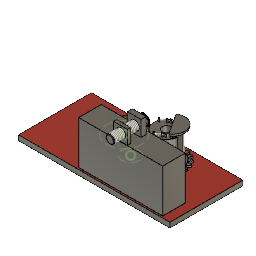
cambio de broca v1 (Autodesk Fusion 360 design; units mm, degrees)
description: Spur Gear; Module: 1.0; Num Teeth: 20; Pressure Angle: 25.0; Backlash: 0.00 mm
description: Spur Gear; Module: 1.0; Num Teeth: 10; Pressure Angle: 25.0; Backlash: 0.00 mm
Autodesk Fusion 360 part; units mm, degrees
(part 1 of 4)
sketch "Boceto1" plane through (0, 0, 0) normal (0, 0, 1) x (1, 0, 0) in component "Spur Gear (20 teeth)"
  circle A0 centre (0, 0) radius 8.7492
  circle A1 centre (0, 0) radius 2.5
extrude "Extruir1" add sketch "Boceto1" along normal blind 1 contours A0 picked at (6.63356, -0.434667) makes body 1 in component "Spur Gear (20 teeth)"
sketch "Boceto2" plane through (0, 0, 0) normal (0, 0, 1) x (1, 0, 0) in component "Spur Gear (20 teeth)"
  spline S0 degree 5 poles (9.009769, -0.981552) (9.015434, -0.98215) (9.026773, -0.983183) (9.043806, -0.984243) (9.066562, -0.984722) (9.095076, -0.984038) (9.123646, -0.982417) (9.152257, -0.980201) (9.1809, -0.977648) (9.209567, -0.974857) (9.238252, -0.971824) (9.266955, -0.968481) (9.295673, -0.964741) (9.324406, -0.960542) (9.353151, -0.955881) (9.381905, -0.950792) (9.410667, -0.945328) (9.439434, -0.939546) (9.468204, -0.933488) (9.496975, -0.927167) (9.525745, -0.920582) (9.554514, -0.913723) (9.583281, -0.906574) (9.612044, -0.899129) (9.640803, -0.891392) (9.669556, -0.883371) (9.698301, -0.875079) (9.727038, -0.86653) (9.755765, -0.857732) (9.784482, -0.848691) (9.813187, -0.839407) (9.84188, -0.829881) (9.870559, -0.820113) (9.899223, -0.810103) (9.927872, -0.799853) (9.956505, -0.789368) (9.985121, -0.778652) (10.013718, -0.767708) (10.042297, -0.756541) (10.070855, -0.745151) (10.099393, -0.733542) (10.127909, -0.721715) (10.156403, -0.709671) (10.184874, -0.697411) (10.213321, -0.684937) (10.241743, -0.672252) (10.270139, -0.659357) (10.298509, -0.646255) (10.326852, -0.632947) (10.355167, -0.619434) (10.383453, -0.605718) (10.41171, -0.591801) (10.439937, -0.577684) (10.468133, -0.563368) (10.496297, -0.548854) (10.524429, -0.534145) (10.552528, -0.51924) (10.580593, -0.504142) (10.608623, -0.488851) (10.636619, -0.47337) (10.664578, -0.457698) (10.692501, -0.441837) (10.720388, -0.425788) (10.748236, -0.409552) (10.776046, -0.393131) (10.803816, -0.376525) (10.831546, -0.359736) (10.859235, -0.342764) (10.886882, -0.325611) (10.914488, -0.308276) (10.942051, -0.290762) (10.964068, -0.276607) (10.980562, -0.26591) (10.991549, -0.258743) (10.99704, -0.25515) knots 0 0 0 0 0 0 0.01428571 0.02857143 0.04285714 0.05714286 0.07142857 0.08571429 0.1 0.11428571 0.12857143 0.14285714 0.15714286 0.17142857 0.18571429 0.2 0.21428571 0.22857143 0.24285714 0.25714286 0.27142857 0.28571429 0.3 0.31428571 0.32857143 0.34285714 0.35714286 0.37142857 0.38571429 0.4 0.41428571 0.42857143 0.44285714 0.45714286 0.47142857 0.48571429 0.5 0.51428571 0.52857143 0.54285714 0.55714286 0.57142857 0.58571429 0.6 0.61428571 0.62857143 0.64285714 0.65714286 0.67142857 0.68571429 0.7 0.71428571 0.72857143 0.74285714 0.75714286 0.77142857 0.78571429 0.8 0.81428571 0.82857143 0.84285714 0.85714286 0.87142857 0.88571429 0.9 0.91428571 0.92857143 0.94285714 0.95714286 0.97142857 0.98571429 1 1 1 1 1 1
  spline S1 degree 5 poles (9.009769, 0.981552) (9.015434, 0.98215) (9.026773, 0.983183) (9.043806, 0.984243) (9.066562, 0.984722) (9.095076, 0.984038) (9.123646, 0.982417) (9.152257, 0.980201) (9.1809, 0.977648) (9.209567, 0.974857) (9.238252, 0.971824) (9.266955, 0.968481) (9.295673, 0.964741) (9.324406, 0.960542) (9.353151, 0.955881) (9.381905, 0.950792) (9.410667, 0.945328) (9.439434, 0.939546) (9.468204, 0.933488) (9.496975, 0.927167) (9.525745, 0.920582) (9.554514, 0.913723) (9.583281, 0.906574) (9.612044, 0.899129) (9.640803, 0.891392) (9.669556, 0.883371) (9.698301, 0.875079) (9.727038, 0.86653) (9.755765, 0.857732) (9.784482, 0.848691) (9.813187, 0.839407) (9.84188, 0.829881) (9.870559, 0.820113) (9.899223, 0.810103) (9.927872, 0.799853) (9.956505, 0.789368) (9.985121, 0.778652) (10.013718, 0.767708) (10.042297, 0.756541) (10.070855, 0.745151) (10.099393, 0.733542) (10.127909, 0.721715) (10.156403, 0.709671) (10.184874, 0.697411) (10.213321, 0.684937) (10.241743, 0.672252) (10.270139, 0.659357) (10.298509, 0.646255) (10.326852, 0.632947) (10.355167, 0.619434) (10.383453, 0.605718) (10.41171, 0.591801) (10.439937, 0.577684) (10.468133, 0.563368) (10.496297, 0.548854) (10.524429, 0.534145) (10.552528, 0.51924) (10.580593, 0.504142) (10.608623, 0.488851) (10.636619, 0.47337) (10.664578, 0.457698) (10.692501, 0.441837) (10.720388, 0.425788) (10.748236, 0.409552) (10.776046, 0.393131) (10.803816, 0.376525) (10.831546, 0.359736) (10.859235, 0.342764) (10.886882, 0.325611) (10.914488, 0.308276) (10.942051, 0.290762) (10.964068, 0.276607) (10.980562, 0.26591) (10.991549, 0.258743) (10.99704, 0.25515) knots 0 0 0 0 0 0 0.01428571 0.02857143 0.04285714 0.05714286 0.07142857 0.08571429 0.1 0.11428571 0.12857143 0.14285714 0.15714286 0.17142857 0.18571429 0.2 0.21428571 0.22857143 0.24285714 0.25714286 0.27142857 0.28571429 0.3 0.31428571 0.32857143 0.34285714 0.35714286 0.37142857 0.38571429 0.4 0.41428571 0.42857143 0.44285714 0.45714286 0.47142857 0.48571429 0.5 0.51428571 0.52857143 0.54285714 0.55714286 0.57142857 0.58571429 0.6 0.61428571 0.62857143 0.64285714 0.65714286 0.67142857 0.68571429 0.7 0.71428571 0.72857143 0.74285714 0.75714286 0.77142857 0.78571429 0.8 0.81428571 0.82857143 0.84285714 0.85714286 0.87142857 0.88571429 0.9 0.91428571 0.92857143 0.94285714 0.95714286 0.97142857 0.98571429 1 1 1 1 1 1
  arc A0 (10.99704, -0.25515) -> (10.99704, 0.25515) centre (0, 0) ccw
  line L0 (8.687796, -0.947559) -> (9.009769, -0.981552)
  line L1 (8.687796, 0.947559) -> (9.009769, 0.981552)
  line L2 (8.687796, -0.947559) -> (8.687796, 0.947559)
  point P0 (9.149052, -0.980379)
  point P1 (9.289749, -0.965437)
  point P2 (9.431291, -0.941141)
  point P3 (9.573428, -0.908982)
  point P4 (9.715981, -0.869786)
  point P5 (9.858805, -0.824084)
  point P6 (10.00177, -0.772251)
  point P7 (10.144756, -0.714565)
  point P8 (10.28765, -0.651241)
  point P9 (10.430344, -0.582452)
  point P10 (10.572732, -0.508339)
  point P11 (10.714711, -0.42902)
  point P12 (10.856181, -0.344594)
  point P13 (9.149052, 0.980379)
  point P14 (9.289749, 0.965437)
  point P15 (9.431291, 0.941141)
  point P16 (9.573428, 0.908982)
  point P17 (9.715981, 0.869786)
  point P18 (9.858805, 0.824084)
  point P19 (10.00177, 0.772251)
  point P20 (10.144756, 0.714565)
  point P21 (10.28765, 0.651241)
  point P22 (10.430344, 0.582452)
  point P23 (10.572732, 0.508339)
  point P24 (10.714711, 0.42902)
  point P25 (10.856181, 0.344594)
extrude "Extruir2" add sketch "Boceto2" along normal blind 1 contours S0 S1 A0 L0 L1 L2 picked at (9.651017, 0.26303) bodies 1 in component "Spur Gear (20 teeth)"
pattern_circular "Patrón C1" count 20 over 360 about axis through (0, 0, 0) along (0, 0, 1) of "Extruir2" in component "Spur Gear (20 teeth)"
sketch "Boceto3" plane through (0, 0, 0) normal (0, 0, 1) x (1, 0, 0) in component "Spur Gear (20 teeth)"
  circle A0 centre (0, 0) radius 10 construction
sketch "Boceto1 (2)" plane through (0, 0, 0) normal (0, 0, 1) x (1, 0, 0) in component "Spur Gear (20 teeth) (1)"
  circle A0 centre (0, 0) radius 8.652617
  circle A1 centre (0, 0) radius 2.130605
extrude "Extruir1'" add sketch "Boceto1 (2)" along normal blind 1 separate body contours A0 picked at (6.446398, -0.429869) makes body 2 in component "Spur Gear (20 teeth) (1)"
sketch "Boceto2 (2)" plane through (0, 0, 0) normal (0, 0, 1) x (1, 0, 0) in component "Spur Gear (20 teeth) (1)"
  spline S0 degree 5 poles (9.009769, -0.981552) (9.015434, -0.98215) (9.026773, -0.983183) (9.043806, -0.984243) (9.066562, -0.984722) (9.095076, -0.984038) (9.123646, -0.982417) (9.152257, -0.980201) (9.1809, -0.977648) (9.209567, -0.974857) (9.238252, -0.971824) (9.266955, -0.968481) (9.295673, -0.964741) (9.324406, -0.960542) (9.353151, -0.955881) (9.381905, -0.950792) (9.410667, -0.945328) (9.439434, -0.939546) (9.468204, -0.933488) (9.496975, -0.927167) (9.525745, -0.920582) (9.554514, -0.913723) (9.583281, -0.906574) (9.612044, -0.899129) (9.640803, -0.891392) (9.669556, -0.883371) (9.698301, -0.875079) (9.727038, -0.86653) (9.755765, -0.857732) (9.784482, -0.848691) (9.813187, -0.839407) (9.84188, -0.829881) (9.870559, -0.820113) (9.899223, -0.810103) (9.927872, -0.799853) (9.956505, -0.789368) (9.985121, -0.778652) (10.013718, -0.767708) (10.042297, -0.756541) (10.070855, -0.745151) (10.099393, -0.733542) (10.127909, -0.721715) (10.156403, -0.709671) (10.184874, -0.697411) (10.213321, -0.684937) (10.241743, -0.672252) (10.270139, -0.659357) (10.298509, -0.646255) (10.326852, -0.632947) (10.355167, -0.619434) (10.383453, -0.605718) (10.41171, -0.591801) (10.439937, -0.577684) (10.468133, -0.563368) (10.496297, -0.548854) (10.524429, -0.534145) (10.552528, -0.51924) (10.580593, -0.504142) (10.608623, -0.488851) (10.636619, -0.47337) (10.664578, -0.457698) (10.692501, -0.441837) (10.720388, -0.425788) (10.748236, -0.409552) (10.776046, -0.393131) (10.803816, -0.376525) (10.831546, -0.359736) (10.859235, -0.342764) (10.886882, -0.325611) (10.914488, -0.308276) (10.942051, -0.290762) (10.964068, -0.276607) (10.980562, -0.26591) (10.991549, -0.258743) (10.99704, -0.25515) knots 0 0 0 0 0 0 0.01428571 0.02857143 0.04285714 0.05714286 0.07142857 0.08571429 0.1 0.11428571 0.12857143 0.14285714 0.15714286 0.17142857 0.18571429 0.2 0.21428571 0.22857143 0.24285714 0.25714286 0.27142857 0.28571429 0.3 0.31428571 0.32857143 0.34285714 0.35714286 0.37142857 0.38571429 0.4 0.41428571 0.42857143 0.44285714 0.45714286 0.47142857 0.48571429 0.5 0.51428571 0.52857143 0.54285714 0.55714286 0.57142857 0.58571429 0.6 0.61428571 0.62857143 0.64285714 0.65714286 0.67142857 0.68571429 0.7 0.71428571 0.72857143 0.74285714 0.75714286 0.77142857 0.78571429 0.8 0.81428571 0.82857143 0.84285714 0.85714286 0.87142857 0.88571429 0.9 0.91428571 0.92857143 0.94285714 0.95714286 0.97142857 0.98571429 1 1 1 1 1 1
  spline S1 degree 5 poles (9.009769, 0.981552) (9.015434, 0.98215) (9.026773, 0.983183) (9.043806, 0.984243) (9.066562, 0.984722) (9.095076, 0.984038) (9.123646, 0.982417) (9.152257, 0.980201) (9.1809, 0.977648) (9.209567, 0.974857) (9.238252, 0.971824) (9.266955, 0.968481) (9.295673, 0.964741) (9.324406, 0.960542) (9.353151, 0.955881) (9.381905, 0.950792) (9.410667, 0.945328) (9.439434, 0.939546) (9.468204, 0.933488) (9.496975, 0.927167) (9.525745, 0.920582) (9.554514, 0.913723) (9.583281, 0.906574) (9.612044, 0.899129) (9.640803, 0.891392) (9.669556, 0.883371) (9.698301, 0.875079) (9.727038, 0.86653) (9.755765, 0.857732) (9.784482, 0.848691) (9.813187, 0.839407) (9.84188, 0.829881) (9.870559, 0.820113) (9.899223, 0.810103) (9.927872, 0.799853) (9.956505, 0.789368) (9.985121, 0.778652) (10.013718, 0.767708) (10.042297, 0.756541) (10.070855, 0.745151) (10.099393, 0.733542) (10.127909, 0.721715) (10.156403, 0.709671) (10.184874, 0.697411) (10.213321, 0.684937) (10.241743, 0.672252) (10.270139, 0.659357) (10.298509, 0.646255) (10.326852, 0.632947) (10.355167, 0.619434) (10.383453, 0.605718) (10.41171, 0.591801) (10.439937, 0.577684) (10.468133, 0.563368) (10.496297, 0.548854) (10.524429, 0.534145) (10.552528, 0.51924) (10.580593, 0.504142) (10.608623, 0.488851) (10.636619, 0.47337) (10.664578, 0.457698) (10.692501, 0.441837) (10.720388, 0.425788) (10.748236, 0.409552) (10.776046, 0.393131) (10.803816, 0.376525) (10.831546, 0.359736) (10.859235, 0.342764) (10.886882, 0.325611) (10.914488, 0.308276) (10.942051, 0.290762) (10.964068, 0.276607) (10.980562, 0.26591) (10.991549, 0.258743) (10.99704, 0.25515) knots 0 0 0 0 0 0 0.01428571 0.02857143 0.04285714 0.05714286 0.07142857 0.08571429 0.1 0.11428571 0.12857143 0.14285714 0.15714286 0.17142857 0.18571429 0.2 0.21428571 0.22857143 0.24285714 0.25714286 0.27142857 0.28571429 0.3 0.31428571 0.32857143 0.34285714 0.35714286 0.37142857 0.38571429 0.4 0.41428571 0.42857143 0.44285714 0.45714286 0.47142857 0.48571429 0.5 0.51428571 0.52857143 0.54285714 0.55714286 0.57142857 0.58571429 0.6 0.61428571 0.62857143 0.64285714 0.65714286 0.67142857 0.68571429 0.7 0.71428571 0.72857143 0.74285714 0.75714286 0.77142857 0.78571429 0.8 0.81428571 0.82857143 0.84285714 0.85714286 0.87142857 0.88571429 0.9 0.91428571 0.92857143 0.94285714 0.95714286 0.97142857 0.98571429 1 1 1 1 1 1
  arc A0 (10.99704, -0.25515) -> (10.99704, 0.25515) centre (0, 0) ccw
  line L0 (8.687796, -0.947559) -> (9.009769, -0.981552)
  line L1 (8.687796, 0.947559) -> (9.009769, 0.981552)
  line L2 (8.687796, -0.947559) -> (8.687796, 0.947559)
  point P0 (9.149052, -0.980379)
  point P1 (9.289749, -0.965437)
  point P2 (9.431291, -0.941141)
  point P3 (9.573428, -0.908982)
  point P4 (9.715981, -0.869786)
  point P5 (9.858805, -0.824084)
  point P6 (10.00177, -0.772251)
  point P7 (10.144756, -0.714565)
  point P8 (10.28765, -0.651241)
  point P9 (10.430344, -0.582452)
  point P10 (10.572732, -0.508339)
  point P11 (10.714711, -0.42902)
  point P12 (10.856181, -0.344594)
  point P13 (9.149052, 0.980379)
  point P14 (9.289749, 0.965437)
  point P15 (9.431291, 0.941141)
  point P16 (9.573428, 0.908982)
  point P17 (9.715981, 0.869786)
  point P18 (9.858805, 0.824084)
  point P19 (10.00177, 0.772251)
  point P20 (10.144756, 0.714565)
  point P21 (10.28765, 0.651241)
  point P22 (10.430344, 0.582452)
  point P23 (10.572732, 0.508339)
  point P24 (10.714711, 0.42902)
  point P25 (10.856181, 0.344594)
extrude "Extruir2'" add sketch "Boceto2 (2)" along normal blind 1 contours S0 S1 A0 L0 L1 L2 picked at (9.651017, 0.26303) bodies 2 makes body 3 in component "Spur Gear (20 teeth) (1)"
pattern_circular "Patrón C1'" count 20 over 360 about axis through (0, 0, 0) along (0, 0, 1) of "Extruir2'" makes body 4 at (9.124655, 3.236379, 0) makes body 5 at (8.336217, 5.821084, 0) makes body 6 at (5.821084, 8.336217, 0) makes body 7 at (2.745052, 9.284296, 0) makes body 8 at (-0.26303, 9.651017, 0) makes body 9 at (-3.236379, 9.124655, 0) makes body 10 at (-5.821084, 8.336217, 0) makes body 11 at (-8.336217, 5.821084, 0) makes body 12 at (-9.124655, 3.236379, 0) makes body 13 at (-9.651017, 0.26303, 0) makes body 14 at (-9.124655, -3.236379, 0) makes body 15 at (-8.336217, -5.821084, 0) makes body 16 at (-5.821084, -8.336217, 0) makes body 17 at (-2.745052, -9.284296, 0) makes body 18 at (-0.26303, -9.651017, 0) makes body 19 at (3.236379, -9.124655, 0) makes body 20 at (5.821084, -8.336217, 0) makes body 21 at (8.336217, -5.821084, 0) makes body 22 at (9.124655, -3.236379, 0) in component "Spur Gear (20 teeth) (1)"
sketch "Boceto3 (2)" plane through (0, 0, 0) normal (0, 0, 1) x (1, 0, 0) in component "Spur Gear (20 teeth) (1)"
  circle A0 centre (0, 0) radius 10 construction
sketch "Boceto1 (3)" plane through (0, 0, 0) normal (0, 0, 1) x (1, 0, 0) in component "Spur Gear (10 teeth)"
  circle A0 centre (0, 0) radius 3.7492
  circle A1 centre (0, 0) radius 2.5
extrude "Extruir1''" add sketch "Boceto1 (3)" along normal blind 1 separate body contours A0 picked at (3.309534, -0.310465) makes body 23 in component "Spur Gear (10 teeth)"
sketch "Boceto2 (3)" plane through (0, 0, 0) normal (0, 0, 1) x (1, 0, 0) in component "Spur Gear (10 teeth)"
  spline S0 degree 5 poles (4.452492, -0.842712) (4.456778, -0.843513) (4.465368, -0.844959) (4.478308, -0.846658) (4.495667, -0.848029) (4.517513, -0.84852) (4.539475, -0.848123) (4.561519, -0.847169) (4.583618, -0.845902) (4.605758, -0.844413) (4.627935, -0.842691) (4.650149, -0.840666) (4.672403, -0.838252) (4.694698, -0.835389) (4.717032, -0.832077) (4.739399, -0.828348) (4.761794, -0.824255) (4.78421, -0.819854) (4.806643, -0.81518) (4.82909, -0.810246) (4.851548, -0.805049) (4.874017, -0.799576) (4.896496, -0.793813) (4.918983, -0.787755) (4.941478, -0.781403) (4.963977, -0.774769) (4.986478, -0.767862) (5.008978, -0.760696) (5.031476, -0.753279) (5.053969, -0.745614) (5.076456, -0.737703) (5.098935, -0.729545) (5.121406, -0.721139) (5.143866, -0.712486) (5.166315, -0.703588) (5.18875, -0.694449) (5.211169, -0.685073) (5.233572, -0.675463) (5.255956, -0.665621) (5.278321, -0.655551) (5.300664, -0.645254) (5.322984, -0.63473) (5.345281, -0.623981) (5.367552, -0.613009) (5.389796, -0.601814) (5.412013, -0.590399) (5.434199, -0.578766) (5.456355, -0.566916) (5.478479, -0.554851) (5.500569, -0.542572) (5.522624, -0.530081) (5.544643, -0.517378) (5.566625, -0.504466) (5.588569, -0.491345) (5.610472, -0.478016) (5.632335, -0.464481) (5.654155, -0.450741) (5.675931, -0.436797) (5.697662, -0.42265) (5.719348, -0.408302) (5.740987, -0.393754) (5.762577, -0.379005) (5.784119, -0.364059) (5.80561, -0.348914) (5.827049, -0.333574) (5.848434, -0.318038) (5.869765, -0.302308) (5.89104, -0.286386) (5.912257, -0.270271) (5.933417, -0.253964) (5.95452, -0.237467) (5.971355, -0.224117) (5.983956, -0.21402) (5.992344, -0.20725) (5.996536, -0.203855) knots 0 0 0 0 0 0 0.01428571 0.02857143 0.04285714 0.05714286 0.07142857 0.08571429 0.1 0.11428571 0.12857143 0.14285714 0.15714286 0.17142857 0.18571429 0.2 0.21428571 0.22857143 0.24285714 0.25714286 0.27142857 0.28571429 0.3 0.31428571 0.32857143 0.34285714 0.35714286 0.37142857 0.38571429 0.4 0.41428571 0.42857143 0.44285714 0.45714286 0.47142857 0.48571429 0.5 0.51428571 0.52857143 0.54285714 0.55714286 0.57142857 0.58571429 0.6 0.61428571 0.62857143 0.64285714 0.65714286 0.67142857 0.68571429 0.7 0.71428571 0.72857143 0.74285714 0.75714286 0.77142857 0.78571429 0.8 0.81428571 0.82857143 0.84285714 0.85714286 0.87142857 0.88571429 0.9 0.91428571 0.92857143 0.94285714 0.95714286 0.97142857 0.98571429 1 1 1 1 1 1
  spline S1 degree 5 poles (4.452492, 0.842712) (4.456778, 0.843513) (4.465368, 0.844959) (4.478308, 0.846658) (4.495667, 0.848029) (4.517513, 0.84852) (4.539475, 0.848123) (4.561519, 0.847169) (4.583618, 0.845902) (4.605758, 0.844413) (4.627935, 0.842691) (4.650149, 0.840666) (4.672403, 0.838252) (4.694698, 0.835389) (4.717032, 0.832077) (4.739399, 0.828348) (4.761794, 0.824255) (4.78421, 0.819854) (4.806643, 0.81518) (4.82909, 0.810246) (4.851548, 0.805049) (4.874017, 0.799576) (4.896496, 0.793813) (4.918983, 0.787755) (4.941478, 0.781403) (4.963977, 0.774769) (4.986478, 0.767862) (5.008978, 0.760696) (5.031476, 0.753279) (5.053969, 0.745614) (5.076456, 0.737703) (5.098935, 0.729545) (5.121406, 0.721139) (5.143866, 0.712486) (5.166315, 0.703588) (5.18875, 0.694449) (5.211169, 0.685073) (5.233572, 0.675463) (5.255956, 0.665621) (5.278321, 0.655551) (5.300664, 0.645254) (5.322984, 0.63473) (5.345281, 0.623981) (5.367552, 0.613009) (5.389796, 0.601814) (5.412013, 0.590399) (5.434199, 0.578766) (5.456355, 0.566916) (5.478479, 0.554851) (5.500569, 0.542572) (5.522624, 0.530081) (5.544643, 0.517378) (5.566625, 0.504466) (5.588569, 0.491345) (5.610472, 0.478016) (5.632335, 0.464481) (5.654155, 0.450741) (5.675931, 0.436797) (5.697662, 0.42265) (5.719348, 0.408302) (5.740987, 0.393754) (5.762577, 0.379005) (5.784119, 0.364059) (5.80561, 0.348914) (5.827049, 0.333574) (5.848434, 0.318038) (5.869765, 0.302308) (5.89104, 0.286386) (5.912257, 0.270271) (5.933417, 0.253964) (5.95452, 0.237467) (5.971355, 0.224117) (5.983956, 0.21402) (5.992344, 0.20725) (5.996536, 0.203855) knots 0 0 0 0 0 0 0.01428571 0.02857143 0.04285714 0.05714286 0.07142857 0.08571429 0.1 0.11428571 0.12857143 0.14285714 0.15714286 0.17142857 0.18571429 0.2 0.21428571 0.22857143 0.24285714 0.25714286 0.27142857 0.28571429 0.3 0.31428571 0.32857143 0.34285714 0.35714286 0.37142857 0.38571429 0.4 0.41428571 0.42857143 0.44285714 0.45714286 0.47142857 0.48571429 0.5 0.51428571 0.52857143 0.54285714 0.55714286 0.57142857 0.58571429 0.6 0.61428571 0.62857143 0.64285714 0.65714286 0.67142857 0.68571429 0.7 0.71428571 0.72857143 0.74285714 0.75714286 0.77142857 0.78571429 0.8 0.81428571 0.82857143 0.84285714 0.85714286 0.87142857 0.88571429 0.9 0.91428571 0.92857143 0.94285714 0.95714286 0.97142857 0.98571429 1 1 1 1 1 1
  arc A0 (5.996536, -0.203855) -> (5.996536, 0.203855) centre (0, 0) ccw
  line L0 (3.673974, -0.697224) -> (4.452492, -0.842712)
  line L1 (3.673974, 0.697224) -> (4.452492, 0.842712)
  line L2 (3.673974, -0.697224) -> (3.673974, 0.697224)
  point P0 (4.558361, -0.847244)
  point P1 (4.666528, -0.838823)
  point P2 (4.776089, -0.821411)
  point P3 (4.886644, -0.796302)
  point P4 (4.997904, -0.764191)
  point P5 (5.109629, -0.725513)
  point P6 (5.221605, -0.680566)
  point P7 (5.333632, -0.629567)
  point P8 (5.445519, -0.572682)
  point P9 (5.557082, -0.510042)
  point P10 (5.668142, -0.441753)
  point P11 (5.77852, -0.367908)
  point P12 (5.888042, -0.288584)
  point P13 (4.558361, 0.847244)
  point P14 (4.666528, 0.838823)
  point P15 (4.776089, 0.821411)
  point P16 (4.886644, 0.796302)
  point P17 (4.997904, 0.764191)
  point P18 (5.109629, 0.725513)
  point P19 (5.221605, 0.680566)
  point P20 (5.333632, 0.629567)
  point P21 (5.445519, 0.572682)
  point P22 (5.557082, 0.510042)
  point P23 (5.668142, 0.441753)
  point P24 (5.77852, 0.367908)
  point P25 (5.888042, 0.288584)
extrude "Extruir2''" add sketch "Boceto2 (3)" along normal blind 1 contours S0 S1 A0 L0 L1 L2 picked at (4.192986, -0.232408) bodies 23 in component "Spur Gear (10 teeth)"
pattern_circular "Patrón C1''" count 10 over 360 about axis through (0, 0, 0) along (0, 0, 1) of "Extruir2''" in component "Spur Gear (10 teeth)"
sketch "Boceto3 (3)" plane through (0, 0, 0) normal (0, 0, 1) x (1, 0, 0) in component "Spur Gear (10 teeth)"
  circle A0 centre (0, 0) radius 5 construction
sketch "Boceto3 (4)" plane through (0, 0, 0) normal (0, 0, 1) x (1, 0, 0)
  line L0 (-43.868107, 21.148143) -> (43.868107, 21.148143)
  line L1 (43.868107, 21.148143) -> (43.868107, -21.148143)
  line L2 (43.868107, -21.148143) -> (-43.868107, -21.148143)
  line L3 (-43.868107, -21.148143) -> (-43.868107, 21.148143)
  line L4 (1.75, 0) -> (22.5, 0)
  line L5 (0, 1.75) -> (0, 22.5)
  constraint horizontal L0
  constraint vertical L1
  constraint horizontal L2
  constraint vertical L3
  constraint symmetric L0 L2 L4
  constraint symmetric L1 L3 L5
extrude "Extruir1'''" add sketch "Boceto3 (4)" along normal blind 3 separate body contours L0 L1 L2 L3 picked at (0, -7.049381) makes body 24
sketch "Boceto4" plane through (0, 0, 3) normal (0, 0, 1) x (-1, 0, 0)
  line L0 (43.868107, 21.148143) -> (-43.868107, 21.148143)
  line L1 (-43.868107, 21.148143) -> (-43.868107, -21.148143)
  line L2 (-43.868107, -21.148143) -> (43.868107, -21.148143)
  line L3 (43.868107, -21.148143) -> (43.868107, 21.148143)
  circle A0 centre (12.332883, -8.53815) radius 2
  circle A1 centre (-12.332883, -8.53815) radius 2
  circle A2 centre (0, 0) radius 2
  line L4 (0, -1.75) -> (0, -22.5)
  line L5 (0, 0) -> (12.332883, -8.53815) construction
  line L6 (0, 0) -> (-12.332883, -8.53815) construction
  dimension "d134" = 4
  dimension "d135" = 4
  dimension "d136" = 4
  dimension "d151" = 15
  constraint coincident A2.centre L5.start
  constraint symmetric A0 A1 L4
  measures "d134" diameter of A0
  measures "d135" diameter of A1
  measures "d136" diameter of A2
extrude "Extruir2'''" add sketch "Boceto4" along normal blind 9 contours A0 | A1 | A2 picked at (12.905881, -9.010838) picked at (-12.969931, -8.156141) picked at (0.668853, -0.773109) bodies 24
sketch "Boceto5" plane through (0, 0, 4) normal (0, 0, 1) x (-1, 0.00000002, 0)
  line L0 (-16.302899, -16.32369) -> (-16.448979, -16.612624)
  spline S0 degree 5 poles (-16.448979, -16.612624) (-16.451549, -16.617708) (-16.456541, -16.627942) (-16.463577, -16.643489) (-16.472104, -16.664593) (-16.481587, -16.691493) (-16.490214, -16.718777) (-16.4983, -16.746311) (-16.506081, -16.773995) (-16.513648, -16.801785) (-16.520996, -16.829679) (-16.528061, -16.857699) (-16.534759, -16.885874) (-16.541034, -16.914226) (-16.546881, -16.942753) (-16.552331, -16.971442) (-16.557433, -17.00027) (-16.56224, -17.029216) (-16.56679, -17.058262) (-16.571094, -17.087403) (-16.575152, -17.116637) (-16.578953, -17.145968) (-16.582482, -17.175399) (-16.585733, -17.204931) (-16.588709, -17.234563) (-16.591418, -17.264291) (-16.593871, -17.294107) (-16.59608, -17.324008) (-16.598053, -17.353987) (-16.599795, -17.384043) (-16.601306, -17.414174) (-16.602587, -17.44438) (-16.603636, -17.474658) (-16.604454, -17.50501) (-16.605042, -17.535431) (-16.605405, -17.565921) (-16.605545, -17.596477) (-16.605467, -17.627097) (-16.605172, -17.657779) (-16.604663, -17.68852) (-16.603941, -17.71932) (-16.603007, -17.750178) (-16.601862, -17.781092) (-16.600508, -17.81206) (-16.598946, -17.843082) (-16.597177, -17.874156) (-16.595202, -17.905281) (-16.593025, -17.936454) (-16.590645, -17.967675) (-16.588064, -17.998943) (-16.585284, -18.030256) (-16.582304, -18.061613) (-16.579127, -18.093013) (-16.575753, -18.124454) (-16.572183, -18.155937) (-16.568418, -18.187458) (-16.56446, -18.219018) (-16.560308, -18.250615) (-16.555964, -18.282248) (-16.551429, -18.313916) (-16.546704, -18.345618) (-16.541789, -18.377353) (-16.536685, -18.40912) (-16.531393, -18.440918) (-16.525914, -18.472746) (-16.520248, -18.504603) (-16.514396, -18.536487) (-16.50836, -18.568398) (-16.502138, -18.600333) (-16.495733, -18.632294) (-16.489145, -18.66428) (-16.483728, -18.689888) (-16.479583, -18.709105) (-16.476783, -18.721921) (-16.475374, -18.72833) knots 0 0 0 0 0 0 0.01428571 0.02857143 0.04285714 0.05714286 0.07142857 0.08571429 0.1 0.11428571 0.12857143 0.14285714 0.15714286 0.17142857 0.18571429 0.2 0.21428571 0.22857143 0.24285714 0.25714286 0.27142857 0.28571429 0.3 0.31428571 0.32857143 0.34285714 0.35714286 0.37142857 0.38571429 0.4 0.41428571 0.42857143 0.44285714 0.45714286 0.47142857 0.48571429 0.5 0.51428571 0.52857143 0.54285714 0.55714286 0.57142857 0.58571429 0.6 0.61428571 0.62857143 0.64285714 0.65714286 0.67142857 0.68571429 0.7 0.71428571 0.72857143 0.74285714 0.75714286 0.77142857 0.78571429 0.8 0.81428571 0.82857143 0.84285714 0.85714286 0.87142857 0.88571429 0.9 0.91428571 0.92857143 0.94285714 0.95714286 0.97142857 0.98571429 1 1 1 1 1 1
  arc A0 (-16.475374, -18.72833) -> (-15.998311, -18.909487) centre (-12.332883, -8.53815) ccw
  spline S1 degree 5 poles (-14.613739, -17.309528) (-14.615191, -17.315037) (-14.618251, -17.326004) (-14.623307, -17.342303) (-14.630938, -17.363748) (-14.6417, -17.390161) (-14.653358, -17.416294) (-14.665586, -17.442256) (-14.678141, -17.468127) (-14.690927, -17.493935) (-14.703946, -17.519676) (-14.71726, -17.545322) (-14.730952, -17.570842) (-14.745077, -17.596213) (-14.759639, -17.621431) (-14.774605, -17.646506) (-14.789924, -17.671455) (-14.805541, -17.696295) (-14.821418, -17.72104) (-14.837541, -17.745693) (-14.85391, -17.770252) (-14.870536, -17.794712) (-14.887431, -17.819068) (-14.904602, -17.843315) (-14.922045, -17.867453) (-14.939751, -17.891486) (-14.957707, -17.915415) (-14.975901, -17.939245) (-14.994324, -17.962979) (-15.012971, -17.986615) (-15.03184, -18.010155) (-15.050932, -18.033597) (-15.070245, -18.05694) (-15.089779, -18.080184) (-15.109531, -18.103328) (-15.129498, -18.126374) (-15.149675, -18.149322) (-15.170058, -18.172171) (-15.190643, -18.194924) (-15.211429, -18.217579) (-15.232413, -18.240137) (-15.253593, -18.262597) (-15.274969, -18.284959) (-15.296537, -18.307223) (-15.318297, -18.329389) (-15.340245, -18.351456) (-15.362381, -18.373426) (-15.384701, -18.395296) (-15.407205, -18.417068) (-15.429889, -18.438742) (-15.452753, -18.460317) (-15.475795, -18.481793) (-15.499013, -18.50317) (-15.522406, -18.524447) (-15.545973, -18.545624) (-15.569711, -18.566702) (-15.59362, -18.587679) (-15.617698, -18.608556) (-15.641944, -18.629333) (-15.666355, -18.650009) (-15.690932, -18.670584) (-15.715672, -18.691058) (-15.740576, -18.71143) (-15.76564, -18.731701) (-15.790864, -18.75187) (-15.816247, -18.771937) (-15.841787, -18.7919) (-15.867483, -18.81176) (-15.893334, -18.831518) (-15.919339, -18.851171) (-15.945497, -18.870722) (-15.966546, -18.886279) (-15.982402, -18.897901) (-15.993003, -18.905629) (-15.998311, -18.909487) knots 0 0 0 0 0 0 0.01428571 0.02857143 0.04285714 0.05714286 0.07142857 0.08571429 0.1 0.11428571 0.12857143 0.14285714 0.15714286 0.17142857 0.18571429 0.2 0.21428571 0.22857143 0.24285714 0.25714286 0.27142857 0.28571429 0.3 0.31428571 0.32857143 0.34285714 0.35714286 0.37142857 0.38571429 0.4 0.41428571 0.42857143 0.44285714 0.45714286 0.47142857 0.48571429 0.5 0.51428571 0.52857143 0.54285714 0.55714286 0.57142857 0.58571429 0.6 0.61428571 0.62857143 0.64285714 0.65714286 0.67142857 0.68571429 0.7 0.71428571 0.72857143 0.74285714 0.75714286 0.77142857 0.78571429 0.8 0.81428571 0.82857143 0.84285714 0.85714286 0.87142857 0.88571429 0.9 0.91428571 0.92857143 0.94285714 0.95714286 0.97142857 0.98571429 1 1 1 1 1 1
  line L1 (-14.613739, -17.309528) -> (-14.531218, -16.996459)
  line L2 (-13.702728, -17.169441) -> (-13.752373, -17.489375)
  spline S2 degree 5 poles (-13.752373, -17.489375) (-13.753247, -17.495004) (-13.754831, -17.506279) (-13.756719, -17.52324) (-13.758307, -17.545946) (-13.759013, -17.57446) (-13.758787, -17.603074) (-13.757968, -17.63176) (-13.756814, -17.660493) (-13.755423, -17.689261) (-13.753792, -17.718061) (-13.751852, -17.746892) (-13.749516, -17.775759) (-13.746722, -17.804662) (-13.743468, -17.8336) (-13.739786, -17.862568) (-13.73573, -17.891562) (-13.731357, -17.920577) (-13.726708, -17.949608) (-13.721797, -17.978652) (-13.716623, -18.007709) (-13.711173, -18.036779) (-13.705435, -18.06586) (-13.699401, -18.094952) (-13.693074, -18.124053) (-13.686464, -18.153162) (-13.679583, -18.182278) (-13.672445, -18.211397) (-13.665057, -18.240519) (-13.657426, -18.269643) (-13.649552, -18.298766) (-13.641436, -18.327889) (-13.633077, -18.35701) (-13.624476, -18.386128) (-13.615635, -18.415243) (-13.606558, -18.444352) (-13.597249, -18.473456) (-13.587712, -18.502553) (-13.577951, -18.531642) (-13.567967, -18.560722) (-13.557762, -18.589791) (-13.547339, -18.61885) (-13.536697, -18.647897) (-13.52584, -18.676932) (-13.514767, -18.705952) (-13.503483, -18.734959) (-13.491987, -18.76395) (-13.480283, -18.792925) (-13.468372, -18.821882) (-13.456255, -18.850822) (-13.443934, -18.879743) (-13.431411, -18.908645) (-13.418686, -18.937526) (-13.405761, -18.966386) (-13.392638, -18.995224) (-13.379316, -19.02404) (-13.365799, -19.052832) (-13.352086, -19.081599) (-13.33818, -19.110342) (-13.324081, -19.139058) (-13.309791, -19.167748) (-13.29531, -19.196412) (-13.280639, -19.225047) (-13.26578, -19.253653) (-13.250733, -19.28223) (-13.2355, -19.310777) (-13.220082, -19.339292) (-13.20448, -19.367775) (-13.188695, -19.396226) (-13.172727, -19.424643) (-13.156577, -19.453027) (-13.143511, -19.475708) (-13.133631, -19.492703) (-13.127008, -19.504027) (-13.123687, -19.509687) knots 0 0 0 0 0 0 0.01428571 0.02857143 0.04285714 0.05714286 0.07142857 0.08571429 0.1 0.11428571 0.12857143 0.14285714 0.15714286 0.17142857 0.18571429 0.2 0.21428571 0.22857143 0.24285714 0.25714286 0.27142857 0.28571429 0.3 0.31428571 0.32857143 0.34285714 0.35714286 0.37142857 0.38571429 0.4 0.41428571 0.42857143 0.44285714 0.45714286 0.47142857 0.48571429 0.5 0.51428571 0.52857143 0.54285714 0.55714286 0.57142857 0.58571429 0.6 0.61428571 0.62857143 0.64285714 0.65714286 0.67142857 0.68571429 0.7 0.71428571 0.72857143 0.74285714 0.75714286 0.77142857 0.78571429 0.8 0.81428571 0.82857143 0.84285714 0.85714286 0.87142857 0.88571429 0.9 0.91428571 0.92857143 0.94285714 0.95714286 0.97142857 0.98571429 1 1 1 1 1 1
  arc A1 (-13.123687, -19.509687) -> (-12.613993, -19.534557) centre (-12.332883, -8.53815) ccw
  spline S3 degree 5 poles (-11.791601, -17.585049) (-11.79128, -17.590737) (-11.790801, -17.602113) (-11.790573, -17.619177) (-11.791203, -17.64193) (-11.793276, -17.670377) (-11.796288, -17.698833) (-11.799895, -17.727303) (-11.803841, -17.755787) (-11.808026, -17.784283) (-11.812454, -17.812787) (-11.817191, -17.841293) (-11.822326, -17.869795) (-11.827921, -17.898289) (-11.833977, -17.926772) (-11.840462, -17.955245) (-11.847321, -17.983706) (-11.854498, -18.012157) (-11.861952, -18.040597) (-11.869667, -18.069026) (-11.877646, -18.097441) (-11.885899, -18.125842) (-11.894441, -18.154226) (-11.903279, -18.182592) (-11.912409, -18.21094) (-11.921822, -18.239267) (-11.931504, -18.267574) (-11.941444, -18.295861) (-11.951632, -18.324125) (-11.962062, -18.352367) (-11.972734, -18.380586) (-11.983646, -18.40878) (-11.994801, -18.436948) (-12.006196, -18.465091) (-12.01783, -18.493207) (-12.029697, -18.521294) (-12.041796, -18.549354) (-12.05412, -18.577384) (-12.066667, -18.605384) (-12.079435, -18.633354) (-12.092421, -18.661292) (-12.105624, -18.689198) (-12.119043, -18.717071) (-12.132676, -18.74491) (-12.146521, -18.772715) (-12.160576, -18.800485) (-12.174839, -18.828219) (-12.189309, -18.855917) (-12.203983, -18.883577) (-12.218859, -18.9112) (-12.233937, -18.938784) (-12.249215, -18.966329) (-12.264691, -18.993835) (-12.280364, -19.021299) (-12.296233, -19.048723) (-12.312297, -19.076104) (-12.328553, -19.103444) (-12.345001, -19.130739) (-12.361639, -19.157991) (-12.378467, -19.185199) (-12.395483, -19.212362) (-12.412686, -19.239479) (-12.430075, -19.26655) (-12.447648, -19.293574) (-12.465405, -19.32055) (-12.483345, -19.347478) (-12.501466, -19.374357) (-12.519767, -19.401186) (-12.538248, -19.427964) (-12.556906, -19.454692) (-12.575743, -19.481369) (-12.590954, -19.50267) (-12.602443, -19.518622) (-12.610137, -19.529247) (-12.613993, -19.534557) knots 0 0 0 0 0 0 0.01428571 0.02857143 0.04285714 0.05714286 0.07142857 0.08571429 0.1 0.11428571 0.12857143 0.14285714 0.15714286 0.17142857 0.18571429 0.2 0.21428571 0.22857143 0.24285714 0.25714286 0.27142857 0.28571429 0.3 0.31428571 0.32857143 0.34285714 0.35714286 0.37142857 0.38571429 0.4 0.41428571 0.42857143 0.44285714 0.45714286 0.47142857 0.48571429 0.5 0.51428571 0.52857143 0.54285714 0.55714286 0.57142857 0.58571429 0.6 0.61428571 0.62857143 0.64285714 0.65714286 0.67142857 0.68571429 0.7 0.71428571 0.72857143 0.74285714 0.75714286 0.77142857 0.78571429 0.8 0.81428571 0.82857143 0.84285714 0.85714286 0.87142857 0.88571429 0.9 0.91428571 0.92857143 0.94285714 0.95714286 0.97142857 0.98571429 1 1 1 1 1 1
  line L3 (-11.791601, -17.585049) -> (-11.809863, -17.261803)
  line L4 (-10.968467, -17.170301) -> (-10.916818, -17.489917)
  spline S4 degree 5 poles (-10.916818, -17.489917) (-10.915909, -17.495541) (-10.913932, -17.506754) (-10.910486, -17.523468) (-10.90498, -17.545554) (-10.89684, -17.57289) (-10.887782, -17.600033) (-10.87814, -17.627062) (-10.868163, -17.654032) (-10.85795, -17.680963) (-10.847499, -17.707849) (-10.836745, -17.73467) (-10.825603, -17.761402) (-10.814014, -17.788027) (-10.801977, -17.814543) (-10.789524, -17.840956) (-10.776707, -17.867277) (-10.763582, -17.89352) (-10.750189, -17.919694) (-10.736543, -17.945799) (-10.722643, -17.971835) (-10.708477, -17.997798) (-10.694033, -18.023682) (-10.679305, -18.049486) (-10.664295, -18.075208) (-10.649013, -18.10085) (-10.633472, -18.126414) (-10.617684, -18.151902) (-10.601659, -18.177316) (-10.585402, -18.202656) (-10.568914, -18.227921) (-10.552195, -18.25311) (-10.535247, -18.278223) (-10.518068, -18.303258) (-10.500663, -18.328216) (-10.483035, -18.353096) (-10.465188, -18.377898) (-10.447127, -18.402624) (-10.428854, -18.427273) (-10.410372, -18.451844) (-10.391684, -18.476337) (-10.372791, -18.500753) (-10.353695, -18.52509) (-10.334396, -18.549348) (-10.314898, -18.573527) (-10.295202, -18.597626) (-10.27531, -18.621646) (-10.255225, -18.645586) (-10.234949, -18.669446) (-10.214482, -18.693225) (-10.193827, -18.716923) (-10.172986, -18.74054) (-10.151959, -18.764076) (-10.130749, -18.78753) (-10.109356, -18.810901) (-10.087782, -18.834189) (-10.066029, -18.857395) (-10.044098, -18.880517) (-10.02199, -18.903556) (-9.999708, -18.92651) (-9.977251, -18.94938) (-9.954621, -18.972165) (-9.93182, -18.994865) (-9.908848, -19.01748) (-9.885707, -19.040009) (-9.862398, -19.062451) (-9.838923, -19.084806) (-9.815283, -19.107074) (-9.791478, -19.129254) (-9.76751, -19.151346) (-9.74338, -19.17335) (-9.723945, -19.190884) (-9.709296, -19.203994) (-9.699498, -19.212717) (-9.694591, -19.217074) knots 0 0 0 0 0 0 0.01428571 0.02857143 0.04285714 0.05714286 0.07142857 0.08571429 0.1 0.11428571 0.12857143 0.14285714 0.15714286 0.17142857 0.18571429 0.2 0.21428571 0.22857143 0.24285714 0.25714286 0.27142857 0.28571429 0.3 0.31428571 0.32857143 0.34285714 0.35714286 0.37142857 0.38571429 0.4 0.41428571 0.42857143 0.44285714 0.45714286 0.47142857 0.48571429 0.5 0.51428571 0.52857143 0.54285714 0.55714286 0.57142857 0.58571429 0.6 0.61428571 0.62857143 0.64285714 0.65714286 0.67142857 0.68571429 0.7 0.71428571 0.72857143 0.74285714 0.75714286 0.77142857 0.78571429 0.8 0.81428571 0.82857143 0.84285714 0.85714286 0.87142857 0.88571429 0.9 0.91428571 0.92857143 0.94285714 0.95714286 0.97142857 0.98571429 1 1 1 1 1 1
  arc A2 (-9.694591, -19.217074) -> (-9.202157, -19.083222) centre (-12.332883, -8.53815) ccw
  spline S5 degree 5 poles (-9.022448, -16.974997) (-9.020385, -16.980308) (-9.016414, -16.990979) (-9.010924, -17.007137) (-9.004492, -17.028971) (-8.997673, -17.056666) (-8.991744, -17.08466) (-8.986377, -17.112851) (-8.981328, -17.141161) (-8.976502, -17.169556) (-8.971905, -17.198033) (-8.967602, -17.226607) (-8.963678, -17.255301) (-8.960193, -17.284129) (-8.957151, -17.31309) (-8.95452, -17.342173) (-8.952249, -17.371361) (-8.950283, -17.400637) (-8.948583, -17.429988) (-8.947136, -17.45941) (-8.945943, -17.4889) (-8.945016, -17.518461) (-8.944369, -17.548096) (-8.944009, -17.577805) (-8.943932, -17.607586) (-8.94413, -17.637436) (-8.944592, -17.66735) (-8.945304, -17.697323) (-8.946259, -17.727352) (-8.947451, -17.757435) (-8.948881, -17.78757) (-8.950547, -17.817757) (-8.952451, -17.847994) (-8.954592, -17.87828) (-8.956968, -17.908615) (-8.959575, -17.938995) (-8.96241, -17.96942) (-8.96547, -17.999886) (-8.96875, -18.030393) (-8.97225, -18.060939) (-8.975967, -18.091523) (-8.979901, -18.122143) (-8.984049, -18.152799) (-8.988412, -18.183488) (-8.992987, -18.214211) (-8.997773, -18.244965) (-9.002768, -18.275749) (-9.007971, -18.306563) (-9.013379, -18.337404) (-9.018991, -18.368272) (-9.024807, -18.399165) (-9.030825, -18.430083) (-9.037044, -18.461024) (-9.043463, -18.491988) (-9.050081, -18.522973) (-9.056897, -18.553979) (-9.06391, -18.585003) (-9.071118, -18.616046) (-9.07852, -18.647105) (-9.086117, -18.678181) (-9.093906, -18.709273) (-9.101887, -18.740379) (-9.11006, -18.771498) (-9.118422, -18.80263) (-9.126974, -18.833773) (-9.135715, -18.864927) (-9.144643, -18.89609) (-9.153758, -18.927261) (-9.163059, -18.95844) (-9.172545, -18.989625) (-9.182216, -19.020817) (-9.190101, -19.045776) (-9.196097, -19.064498) (-9.200131, -19.076981) (-9.202157, -19.083222) knots 0 0 0 0 0 0 0.01428571 0.02857143 0.04285714 0.05714286 0.07142857 0.08571429 0.1 0.11428571 0.12857143 0.14285714 0.15714286 0.17142857 0.18571429 0.2 0.21428571 0.22857143 0.24285714 0.25714286 0.27142857 0.28571429 0.3 0.31428571 0.32857143 0.34285714 0.35714286 0.37142857 0.38571429 0.4 0.41428571 0.42857143 0.44285714 0.45714286 0.47142857 0.48571429 0.5 0.51428571 0.52857143 0.54285714 0.55714286 0.57142857 0.58571429 0.6 0.61428571 0.62857143 0.64285714 0.65714286 0.67142857 0.68571429 0.7 0.71428571 0.72857143 0.74285714 0.75714286 0.77142857 0.78571429 0.8 0.81428571 0.82857143 0.84285714 0.85714286 0.87142857 0.88571429 0.9 0.91428571 0.92857143 0.94285714 0.95714286 0.97142857 0.98571429 1 1 1 1 1 1
  line L5 (-9.022448, -16.974997) -> (-9.139704, -16.673214)
  line L6 (-8.367765, -16.326186) -> (-8.219877, -16.614198)
  spline S6 degree 5 poles (-8.219877, -16.614198) (-8.217274, -16.619266) (-8.211929, -16.629319) (-8.203487, -16.644151) (-8.191425, -16.663454) (-8.175237, -16.686936) (-8.158234, -16.709953) (-8.140711, -16.732679) (-8.122889, -16.755246) (-8.104854, -16.777703) (-8.086606, -16.800043) (-8.06809, -16.822228) (-8.049233, -16.844209) (-8.029984, -16.865949) (-8.010342, -16.887448) (-7.990336, -16.90872) (-7.970012, -16.929792) (-7.94942, -16.950695) (-7.928595, -16.971449) (-7.90755, -16.99206) (-7.886284, -17.012526) (-7.864789, -17.032841) (-7.843054, -17.052995) (-7.821072, -17.072984) (-7.798848, -17.092809) (-7.776391, -17.112473) (-7.75371, -17.131984) (-7.730819, -17.151346) (-7.707725, -17.170564) (-7.684433, -17.18964) (-7.660945, -17.208573) (-7.637261, -17.227363) (-7.613381, -17.246009) (-7.589307, -17.264511) (-7.565042, -17.282869) (-7.540588, -17.301084) (-7.51595, -17.319157) (-7.491132, -17.337092) (-7.466137, -17.354887) (-7.440967, -17.372545) (-7.415625, -17.390065) (-7.390111, -17.407447) (-7.364429, -17.424691) (-7.338579, -17.441799) (-7.312563, -17.458769) (-7.286384, -17.475603) (-7.260043, -17.4923) (-7.233544, -17.508861) (-7.206886, -17.525287) (-7.180073, -17.541578) (-7.153106, -17.557734) (-7.125987, -17.573755) (-7.098716, -17.589641) (-7.071296, -17.605392) (-7.043728, -17.621009) (-7.016014, -17.636491) (-6.988154, -17.651839) (-6.960152, -17.667052) (-6.932007, -17.682131) (-6.903722, -17.697076) (-6.875297, -17.711888) (-6.846733, -17.726565) (-6.818033, -17.741108) (-6.789197, -17.755517) (-6.760227, -17.769792) (-6.731124, -17.783933) (-6.70189, -17.79794) (-6.672526, -17.811813) (-6.643032, -17.825551) (-6.61341, -17.839156) (-6.583661, -17.852626) (-6.55976, -17.863295) (-6.541777, -17.871237) (-6.529762, -17.876505) (-6.523749, -17.879133) knots 0 0 0 0 0 0 0.01428571 0.02857143 0.04285714 0.05714286 0.07142857 0.08571429 0.1 0.11428571 0.12857143 0.14285714 0.15714286 0.17142857 0.18571429 0.2 0.21428571 0.22857143 0.24285714 0.25714286 0.27142857 0.28571429 0.3 0.31428571 0.32857143 0.34285714 0.35714286 0.37142857 0.38571429 0.4 0.41428571 0.42857143 0.44285714 0.45714286 0.47142857 0.48571429 0.5 0.51428571 0.52857143 0.54285714 0.55714286 0.57142857 0.58571429 0.6 0.61428571 0.62857143 0.64285714 0.65714286 0.67142857 0.68571429 0.7 0.71428571 0.72857143 0.74285714 0.75714286 0.77142857 0.78571429 0.8 0.81428571 0.82857143 0.84285714 0.85714286 0.87142857 0.88571429 0.9 0.91428571 0.92857143 0.94285714 0.95714286 0.97142857 0.98571429 1 1 1 1 1 1
  arc A3 (-6.523749, -17.879133) -> (-6.096779, -17.599662) centre (-12.332883, -8.53815) ccw
  spline S7 degree 5 poles (-6.577343, -15.539088) (-6.57374, -15.543501) (-6.566665, -15.552422) (-6.556451, -15.566093) (-6.543587, -15.584871) (-6.528544, -15.609104) (-6.514254, -15.633895) (-6.500438, -15.659048) (-6.486888, -15.684412) (-6.473524, -15.709926) (-6.460352, -15.735588) (-6.447429, -15.761435) (-6.434831, -15.787512) (-6.422608, -15.813852) (-6.410766, -15.840455) (-6.399276, -15.867301) (-6.388096, -15.894359) (-6.37718, -15.921595) (-6.366493, -15.948985) (-6.356025, -15.976519) (-6.345778, -16.004197) (-6.335762, -16.032025) (-6.325989, -16.060009) (-6.316465, -16.088153) (-6.307189, -16.116453) (-6.298154, -16.144903) (-6.289349, -16.173495) (-6.280764, -16.202222) (-6.272392, -16.231076) (-6.26423, -16.260055) (-6.256277, -16.289157) (-6.248534, -16.318381) (-6.241001, -16.347726) (-6.233678, -16.377192) (-6.226564, -16.406776) (-6.219655, -16.436475) (-6.21295, -16.466287) (-6.206445, -16.496208) (-6.200138, -16.526236) (-6.194027, -16.556368) (-6.188112, -16.586604) (-6.18239, -16.616941) (-6.176863, -16.647378) (-6.171529, -16.677913) (-6.166386, -16.708546) (-6.161434, -16.739274) (-6.156672, -16.770095) (-6.152098, -16.801008) (-6.147711, -16.832011) (-6.14351, -16.863102) (-6.139495, -16.894281) (-6.135664, -16.925545) (-6.132017, -16.956894) (-6.128554, -16.988326) (-6.125273, -17.01984) (-6.122174, -17.051434) (-6.119256, -17.083107) (-6.116519, -17.114857) (-6.113961, -17.146685) (-6.111583, -17.178587) (-6.109383, -17.210564) (-6.107362, -17.242614) (-6.105517, -17.274735) (-6.10385, -17.306928) (-6.10236, -17.33919) (-6.101046, -17.371519) (-6.099907, -17.403916) (-6.098943, -17.436378) (-6.098154, -17.468905) (-6.097539, -17.501495) (-6.097098, -17.534149) (-6.096884, -17.560323) (-6.096801, -17.579982) (-6.096781, -17.5931) (-6.096779, -17.599662) knots 0 0 0 0 0 0 0.01428571 0.02857143 0.04285714 0.05714286 0.07142857 0.08571429 0.1 0.11428571 0.12857143 0.14285714 0.15714286 0.17142857 0.18571429 0.2 0.21428571 0.22857143 0.24285714 0.25714286 0.27142857 0.28571429 0.3 0.31428571 0.32857143 0.34285714 0.35714286 0.37142857 0.38571429 0.4 0.41428571 0.42857143 0.44285714 0.45714286 0.47142857 0.48571429 0.5 0.51428571 0.52857143 0.54285714 0.55714286 0.57142857 0.58571429 0.6 0.61428571 0.62857143 0.64285714 0.65714286 0.67142857 0.68571429 0.7 0.71428571 0.72857143 0.74285714 0.75714286 0.77142857 0.78571429 0.8 0.81428571 0.82857143 0.84285714 0.85714286 0.87142857 0.88571429 0.9 0.91428571 0.92857143 0.94285714 0.95714286 0.97142857 0.98571429 1 1 1 1 1 1
  line L7 (-6.577343, -15.539088) -> (-6.782116, -15.288309)
  line L8 (-6.155196, -14.719723) -> (-5.925545, -14.947939)
  spline S8 degree 5 poles (-5.925545, -14.947939) (-5.921504, -14.951955) (-5.913314, -14.959864) (-5.900702, -14.971361) (-5.883266, -14.985992) (-5.860613, -15.003323) (-5.83733, -15.019959) (-5.813642, -15.036158) (-5.789718, -15.052113) (-5.765626, -15.067897) (-5.741368, -15.083505) (-5.716903, -15.098883) (-5.692176, -15.11396) (-5.667151, -15.128689) (-5.641827, -15.143065) (-5.616227, -15.157114) (-5.590386, -15.170875) (-5.564343, -15.184391) (-5.538124, -15.197694) (-5.511739, -15.210793) (-5.48519, -15.223686) (-5.458469, -15.236364) (-5.43157, -15.248815) (-5.404487, -15.261033) (-5.377225, -15.27302) (-5.349789, -15.284783) (-5.32219, -15.296329) (-5.294436, -15.30767) (-5.266534, -15.318811) (-5.238487, -15.329756) (-5.210297, -15.340504) (-5.181966, -15.351056) (-5.153494, -15.36141) (-5.124881, -15.371567) (-5.09613, -15.381528) (-5.067244, -15.391294) (-5.038227, -15.40087) (-5.009082, -15.410257) (-4.97981, -15.419458) (-4.950416, -15.428473) (-4.9209, -15.437305) (-4.891264, -15.445952) (-4.86151, -15.454416) (-4.831639, -15.462698) (-4.801652, -15.470799) (-4.771552, -15.478719) (-4.741341, -15.486459) (-4.711021, -15.494021) (-4.680592, -15.501406) (-4.650057, -15.508613) (-4.619418, -15.515645) (-4.588675, -15.522501) (-4.55783, -15.529183) (-4.526885, -15.53569) (-4.49584, -15.542023) (-4.464698, -15.548183) (-4.433459, -15.554171) (-4.402126, -15.559987) (-4.370699, -15.565631) (-4.33918, -15.571103) (-4.307569, -15.576406) (-4.275868, -15.581538) (-4.244079, -15.586501) (-4.212201, -15.591294) (-4.180238, -15.595918) (-4.14819, -15.600374) (-4.116058, -15.604661) (-4.083844, -15.608781) (-4.051548, -15.612733) (-4.019173, -15.616518) (-3.986717, -15.620136) (-3.960688, -15.622897) (-3.941131, -15.624893) (-3.928077, -15.626191) (-3.921546, -15.626831) knots 0 0 0 0 0 0 0.01428571 0.02857143 0.04285714 0.05714286 0.07142857 0.08571429 0.1 0.11428571 0.12857143 0.14285714 0.15714286 0.17142857 0.18571429 0.2 0.21428571 0.22857143 0.24285714 0.25714286 0.27142857 0.28571429 0.3 0.31428571 0.32857143 0.34285714 0.35714286 0.37142857 0.38571429 0.4 0.41428571 0.42857143 0.44285714 0.45714286 0.47142857 0.48571429 0.5 0.51428571 0.52857143 0.54285714 0.55714286 0.57142857 0.58571429 0.6 0.61428571 0.62857143 0.64285714 0.65714286 0.67142857 0.68571429 0.7 0.71428571 0.72857143 0.74285714 0.75714286 0.77142857 0.78571429 0.8 0.81428571 0.82857143 0.84285714 0.85714286 0.87142857 0.88571429 0.9 0.91428571 0.92857143 0.94285714 0.95714286 0.97142857 0.98571429 1 1 1 1 1 1
  arc A4 (-3.921546, -15.626831) -> (-3.601835, -15.229098) centre (-12.332883, -8.53815) ccw